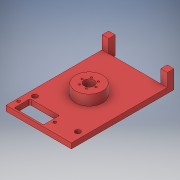
# Autodesk Inventor part: 000.801 - Опора
Saved by Autodesk Inventor 2019 (Build 230136000, 136)
## iProperties
Created: 2020-03-13
Part Number: 000.801 - Опора
Material: Пластик АБС
Document SubType Name: Modeling
Designer: Петров Иван
Density: 1.06 g/cm^3
Appearance: Гладкий — красный
Author: Петров Иван
Autodesk Inventor part; units mm, degrees
ref_plane "YZ Plane" through (0, 0, 0) normal (1, 0, 0) x (0, 1, 0)
ref_plane "XZ Plane" through (0, 0, 0) normal (0, 1, 0) x (-1, 0, 0)
ref_plane "XY Plane" through (0, 0, 0) normal (0, 0, 1) x (1, 0, 0)
sketch "Эскиз1" plane through (0, 0, 0) normal (0, 1, 0) x (-1, 0, 0)
  circle A0 centre (-2.65, -4.5899) radius 0.75
  circle A1 centre (2.65, -4.5899) radius 0.75
  circle A2 centre (5.3, 0) radius 0.75
  circle A3 centre (2.65, 4.5899) radius 0.75
  circle A4 centre (-2.65, 4.5899) radius 0.75
  circle A5 centre (-5.3, 0) radius 0.75
  circle A6 centre (0, 0) radius 3.85
  arc A7 (-3.4059, 8.2225) -> (-3.1756, 6.1003) centre (3.6513, 7.9146) ccw
  arc A8 (-3.1756, 6.1003) -> (-3.6952, 5.8003) centre (0, 0) ccw
  arc A9 (-3.6952, 5.8003) -> (-5.418, 7.0608) centre (-8.6799, 0.7952) ccw
  arc A10 (-5.418, 7.0608) -> (-6.0128, 6.5618) centre (0, 0) ccw
  arc A11 (-6.0128, 6.5618) -> (-5.0705, 4.6463) centre (0.7241, 8.6861) ccw
  arc A12 (-5.0705, 4.6463) -> (-5.4562, 4.1867) centre (0, 0) ccw
  arc A13 (-5.4562, 4.1867) -> (-7.5062, 4.782) centre (-8.4284, -2.2214) ccw
  arc A14 (-7.5062, 4.782) -> (-7.8944, 4.1096) centre (0, 0) ccw
  arc A15 (-7.8944, 4.1096) -> (-6.3539, 2.6319) centre (-2.2904, 8.4099) ccw
  arc A16 (-6.3539, 2.6319) -> (-6.5591, 2.0681) centre (0, 0) ccw
  arc A17 (-6.5591, 2.0681) -> (-8.689, 1.9263) centre (-7.1604, -4.9702) ccw
  arc A18 (-8.689, 1.9263) -> (-8.8239, 1.1617) centre (0, 0) ccw
  arc A19 (-8.8239, 1.1617) -> (-6.8708, 0.3) centre (-5.0286, 7.1194) ccw
  arc A20 (-6.8708, 0.3) -> (-6.8708, -0.3) centre (0, 0) ccw
  arc A21 (-6.8708, -0.3) -> (-8.8239, -1.1617) centre (-5.0286, -7.1194) ccw
  arc A22 (-8.8239, -1.1617) -> (-8.689, -1.9263) centre (0, 0) ccw
  arc A23 (-8.689, -1.9263) -> (-6.5591, -2.0681) centre (-7.1604, 4.9702) ccw
  arc A24 (-6.5591, -2.0681) -> (-6.3539, -2.6319) centre (0, 0) ccw
  arc A25 (-6.3539, -2.6319) -> (-7.8944, -4.1096) centre (-2.2904, -8.4099) ccw
  arc A26 (-7.8944, -4.1096) -> (-7.5062, -4.782) centre (0, 0) ccw
  arc A27 (-7.5062, -4.782) -> (-5.4562, -4.1867) centre (-8.4284, 2.2214) ccw
  arc A28 (-5.4562, -4.1867) -> (-5.0705, -4.6463) centre (0, 0) ccw
  arc A29 (-5.0705, -4.6463) -> (-6.0128, -6.5618) centre (0.7241, -8.6861) ccw
  arc A30 (-6.0128, -6.5618) -> (-5.418, -7.0608) centre (0, 0) ccw
  arc A31 (-5.418, -7.0608) -> (-3.6952, -5.8003) centre (-8.6799, -0.7952) ccw
  arc A32 (-3.6952, -5.8003) -> (-3.1756, -6.1003) centre (0, 0) ccw
  arc A33 (-3.1756, -6.1003) -> (-3.4059, -8.2225) centre (3.6513, -7.9146) ccw
  arc A34 (-3.4059, -8.2225) -> (-2.6763, -8.4881) centre (0, 0) ccw
  arc A35 (-2.6763, -8.4881) -> (-1.4885, -6.7144) centre (-7.8845, -3.716) ccw
  arc A36 (-1.4885, -6.7144) -> (-0.8977, -6.8185) centre (0, 0) ccw
  arc A37 (-0.8977, -6.8185) -> (-0.3882, -8.8915) centre (6.138, -6.1885) ccw
  arc A38 (-0.3882, -8.8915) -> (0.3882, -8.8915) centre (0, 0) ccw
  arc A39 (0.3882, -8.8915) -> (0.8977, -6.8185) centre (-6.138, -6.1885) ccw
  arc A40 (0.8977, -6.8185) -> (1.4885, -6.7144) centre (0, 0) ccw
  arc A41 (1.4885, -6.7144) -> (2.6763, -8.4881) centre (7.8845, -3.716) ccw
  arc A42 (2.6763, -8.4881) -> (3.4059, -8.2225) centre (0, 0) ccw
  arc A43 (3.4059, -8.2225) -> (3.1756, -6.1003) centre (-3.6513, -7.9146) ccw
  arc A44 (3.1756, -6.1003) -> (3.6952, -5.8003) centre (0, 0) ccw
  arc A45 (3.6952, -5.8003) -> (5.418, -7.0608) centre (8.6799, -0.7952) ccw
  arc A46 (5.418, -7.0608) -> (6.0128, -6.5618) centre (0, 0) ccw
  arc A47 (6.0128, -6.5618) -> (5.0705, -4.6463) centre (-0.7241, -8.6861) ccw
  arc A48 (5.0705, -4.6463) -> (5.4562, -4.1867) centre (0, 0) ccw
  arc A49 (5.4562, -4.1867) -> (7.5062, -4.782) centre (8.4284, 2.2214) ccw
  arc A50 (7.5062, -4.782) -> (7.8944, -4.1096) centre (0, 0) ccw
  arc A51 (7.8944, -4.1096) -> (6.3539, -2.6319) centre (2.2904, -8.4099) ccw
  arc A52 (6.3539, -2.6319) -> (6.5591, -2.0681) centre (0, 0) ccw
  arc A53 (6.5591, -2.0681) -> (8.689, -1.9263) centre (7.1604, 4.9702) ccw
  arc A54 (8.689, -1.9263) -> (8.8239, -1.1617) centre (0, 0) ccw
  arc A55 (8.8239, -1.1617) -> (6.8708, -0.3) centre (5.0286, -7.1194) ccw
  arc A56 (6.8708, -0.3) -> (6.8708, 0.3) centre (0, 0) ccw
  arc A57 (6.8708, 0.3) -> (8.8239, 1.1617) centre (5.0286, 7.1194) ccw
  arc A58 (8.8239, 1.1617) -> (8.689, 1.9263) centre (0, 0) ccw
  arc A59 (8.689, 1.9263) -> (6.5591, 2.0681) centre (7.1604, -4.9702) ccw
  arc A60 (6.5591, 2.0681) -> (6.3539, 2.6319) centre (0, 0) ccw
  arc A61 (6.3539, 2.6319) -> (7.8944, 4.1096) centre (2.2904, 8.4099) ccw
  arc A62 (7.8944, 4.1096) -> (7.5062, 4.782) centre (0, 0) ccw
  arc A63 (7.5062, 4.782) -> (5.4562, 4.1867) centre (8.4284, -2.2214) ccw
  arc A64 (5.4562, 4.1867) -> (5.0705, 4.6463) centre (0, 0) ccw
  arc A65 (5.0705, 4.6463) -> (6.0128, 6.5618) centre (-0.7241, 8.6861) ccw
  arc A66 (6.0128, 6.5618) -> (5.418, 7.0608) centre (0, 0) ccw
  arc A67 (5.418, 7.0608) -> (3.6952, 5.8003) centre (8.6799, 0.7952) ccw
  arc A68 (3.6952, 5.8003) -> (3.1756, 6.1003) centre (0, 0) ccw
  arc A69 (3.1756, 6.1003) -> (3.4059, 8.2225) centre (-3.6513, 7.9146) ccw
  arc A70 (3.4059, 8.2225) -> (2.6763, 8.4881) centre (0, 0) ccw
  arc A71 (2.6763, 8.4881) -> (1.4885, 6.7144) centre (7.8845, 3.716) ccw
  arc A72 (1.4885, 6.7144) -> (0.8977, 6.8185) centre (0, 0) ccw
  arc A73 (0.8977, 6.8185) -> (0.3882, 8.8915) centre (-6.138, 6.1885) ccw
  arc A74 (0.3882, 8.8915) -> (-0.3882, 8.8915) centre (0, 0) ccw
  arc A75 (-0.3882, 8.8915) -> (-0.8977, 6.8185) centre (6.138, 6.1885) ccw
  arc A76 (-0.8977, 6.8185) -> (-1.4885, 6.7144) centre (0, 0) ccw
  arc A77 (-1.4885, 6.7144) -> (-2.6763, 8.4881) centre (-7.8845, 3.716) ccw
  arc A78 (-2.6763, 8.4881) -> (-3.4059, 8.2225) centre (0, 0) ccw
  line L0 (-25, 25) -> (25, 25)
  line L1 (25, 25) -> (25, -25)
  line L2 (25, -25) -> (-25, -25)
  line L3 (-25, -25) -> (-25, 25)
  line L4 (-25, 25) -> (25, -25) construction
  line L5 (25, 25) -> (-25, -25) construction
  dimension "d4" = 50
  dimension "d5" = 50
  constraints: 144 point on circle, 79 centre point, 12 end point, 2 midpoint, 2 parallel, 1 horizontal, 1 perpendicular
  measures "d4" distance of L1.end L2.end
  measures "d5" distance of L0.end L1.end
extrude "Выдавливание1" add sketch "Эскиз1" along normal blind 4 contours A78 A77 A76 A75 A74 A73 A72 A71 A70 A69 A68 A67 A66 A65 A64 A63 A62 A61 A60 A59 A58 A57 A56 A55 A54 A53 A52 A51 A50 A49 A48 A47 A46 A45 A44 A43 A42 A41 A40 A39 A38 A37 A36 A35 A34 A33 A32 A31 A30 A29 A28 A27 A26 A25 A24 A23 A22 A21 A20 A19 A18 A17 A16 A15 A14 A13 A12 A11 A10 A9 A8 A7 | L0 L1 L2 L3
sketch "Эскиз2" plane through (0, 4, 0) normal (0, 1, 0) x (1, 0, 0)
  line L0 (-8.6363, -28.2584) -> (-8.5162, -28.2584)
  arc A0 (-8.5162, -34.0584) -> (-8.5162, -28.2584) centre (-8.5162, -31.1584) ccw
  line L1 (-8.5162, -34.0584) -> (-8.6363, -34.0584)
  arc A1 (-12.5542, -37.1584) -> (-8.6363, -34.0584) centre (-14.1162, -31.1584) ccw
  line L2 (-12.5542, -37.1584) -> (1.4338, -37.1584)
  arc A2 (1.4338, -37.1584) -> (2.1838, -36.4084) centre (1.4338, -36.4084) ccw
  line L3 (2.1838, -36.4084) -> (2.1838, -25.9084)
  arc A3 (2.1838, -25.9084) -> (1.4338, -25.1584) centre (1.4338, -25.9084) ccw
  line L4 (1.4338, -25.1584) -> (-12.5542, -25.1584)
  arc A4 (-8.6363, -28.2584) -> (-12.5542, -25.1584) centre (-14.1162, -31.1584) ccw
  line L5 (-4.2162, -36.2584) -> (0.7838, -36.2584)
  arc A5 (-4.7162, -35.7584) -> (-4.2162, -36.2584) centre (-4.2162, -35.7584) ccw
  line L6 (-4.7162, -26.5584) -> (-4.7162, -35.7584)
  arc A6 (-4.2162, -26.0584) -> (-4.7162, -26.5584) centre (-4.2162, -26.5584) ccw
  line L7 (0.7838, -26.0584) -> (-4.2162, -26.0584)
  arc A7 (1.2838, -26.5584) -> (0.7838, -26.0584) centre (0.7838, -26.5584) ccw
  line L8 (1.2838, -35.7584) -> (1.2838, -26.5584)
  arc A8 (0.7838, -36.2584) -> (1.2838, -35.7584) centre (0.7838, -35.7584) ccw
  arc A9 (5.8864, -30.6084) -> (5.8864, -31.7084) centre (4.9338, -31.1584) ccw
  line L9 (7.0838, -30.6084) -> (5.8864, -30.6084)
  line L10 (7.0838, -30.6084) -> (7.0838, -25.9084)
  arc A10 (7.0838, -25.9084) -> (6.2338, -25.0584) centre (6.2338, -25.9084) ccw
  line L11 (6.2338, -25.0584) -> (1.4338, -25.0584)
  arc A11 (2.2838, -25.9084) -> (1.4338, -25.0584) centre (1.4338, -25.9084) ccw
  line L12 (2.2838, -36.4084) -> (2.2838, -25.9084)
  arc A12 (1.4338, -37.2584) -> (2.2838, -36.4084) centre (1.4338, -36.4084) ccw
  line L13 (1.4338, -37.2584) -> (6.2338, -37.2584)
  arc A13 (6.2338, -37.2584) -> (7.0838, -36.4084) centre (6.2338, -36.4084) ccw
  line L14 (7.0838, -36.4084) -> (7.0838, -31.7084)
  line L15 (5.8864, -31.7084) -> (7.0838, -31.7084)
  line L16 (-25.0162, -25.9084) -> (-25.0162, -30.6084)
  line L17 (-23.8188, -30.6084) -> (-25.0162, -30.6084)
  arc A14 (-23.8188, -31.7084) -> (-23.8188, -30.6084) centre (-22.8662, -31.1584) ccw
  line L18 (-25.0162, -31.7084) -> (-23.8188, -31.7084)
  line L19 (-25.0162, -31.7084) -> (-25.0162, -36.4084)
  arc A15 (-25.0162, -36.4084) -> (-24.1662, -37.2584) centre (-24.1662, -36.4084) ccw
  line L20 (-24.1662, -37.2584) -> (-19.3662, -37.2584)
  arc A16 (-20.2162, -36.4084) -> (-19.3662, -37.2584) centre (-19.3662, -36.4084) ccw
  line L21 (-20.2162, -25.9084) -> (-20.2162, -36.4084)
  arc A17 (-19.3662, -25.0584) -> (-20.2162, -25.9084) centre (-19.3662, -25.9084) ccw
  line L22 (-19.3662, -25.0584) -> (-24.1662, -25.0584)
  arc A18 (-24.1662, -25.0584) -> (-25.0162, -25.9084) centre (-24.1662, -25.9084) ccw
  line L23 (-19.3662, -25.0584) -> (-15.6783, -25.0584)
  line L24 (-12.5542, -25.0584) -> (-14.1162, -25.0584)
  line L25 (-14.1162, -25.0584) -> (-15.6783, -25.0584)
  line L26 (-12.5542, -25.0584) -> (1.4338, -25.0584)
  line L27 (1.4338, -37.2584) -> (-12.5542, -37.2584)
  line L28 (-15.6783, -37.2584) -> (-19.3662, -37.2584)
  line L29 (-15.6783, -37.2584) -> (-14.1162, -37.2584)
  line L30 (-14.1162, -37.2584) -> (-12.5542, -37.2584)
  arc A19 (-15.6783, -25.1584) -> (-20.1162, -29.5963) centre (-14.1162, -31.1584) ccw
  line L31 (-15.6783, -25.1584) -> (-19.3662, -25.1584)
  arc A20 (-19.3662, -25.1584) -> (-20.1162, -25.9084) centre (-19.3662, -25.9084) ccw
  line L32 (-20.1162, -25.9084) -> (-20.1162, -29.5963)
  line L33 (-19.3662, -37.1584) -> (-15.6783, -37.1584)
  arc A21 (-20.1162, -32.7204) -> (-15.6783, -37.1584) centre (-14.1162, -31.1584) ccw
  line L34 (-20.1162, -32.7204) -> (-20.1162, -36.4084)
  arc A22 (-20.1162, -36.4084) -> (-19.3662, -37.1584) centre (-19.3662, -36.4084) ccw
  circle A23 centre (4.9338, -31.1584) radius 1.1
  line L35 (5.8864, -30.6084) -> (7.0838, -30.6084)
  line L36 (7.0838, -31.7084) -> (7.0838, -30.6084)
  circle A24 centre (-22.8662, -31.1584) radius 1.1
  line L37 (-25.0162, -30.6084) -> (-23.8188, -30.6084)
  line L38 (-25.0162, -31.7084) -> (-25.0162, -30.6084)
  circle A25 centre (-14.1162, -31.1584) radius 0.8
  line L39 (-25, -25) -> (-25, 25) projected
  line L40 (25, -38.5621) -> (-25, -38.5621)
  line L41 (-25, -38.5621) -> (-25, -25)
  line L42 (-25, -25) -> (25, -25)
  line L43 (25, -25) -> (25, -38.5621)
  point P0 (0, 0)
  point P1 (-8.9662, -31.1584)
  constraints: 86 end point, 46 point on circle, 25 centre point, 2 coincident, 2 parallel, 1 collinear, 1 concentric, 1 horizontal, 1 perpendicular, 1 vertical, 3 other
extrude "Выдавливание2" add sketch "Эскиз2" against normal blind 4 contours A9 L15 L14 A13 L13 A12 L12 A11 L11 A10 L10 L9 | L9 L36 L15 A23 | L10 A10 L11 L26 L24 L25 L23 L22 A18 L41 L42 L43 L40 A15 L20 L28 L29 L30 L27 L13 A13 L14 L36 | A17 L21 A16 L20 A15 L41 L18 A14 L17 A18 L22 | L17 A24 L18 L41
sketch "Эскиз3" plane through (0, 4, 0) normal (0, 1, 0) x (1, 0, 0)
  circle A0 centre (-2.65, -4.5899) radius 0.75
  circle A1 centre (2.65, -4.5899) radius 0.75
  circle A2 centre (5.3, 0) radius 0.75
  circle A3 centre (2.65, 4.5899) radius 0.75
  circle A4 centre (-2.65, 4.5899) radius 0.75
  circle A5 centre (-5.3, 0) radius 0.75
  circle A6 centre (0, 0) radius 3.85
  arc A7 (-3.4059, 8.2225) -> (-3.1756, 6.1003) centre (3.6513, 7.9146) ccw
  arc A8 (-3.1756, 6.1003) -> (-3.6952, 5.8003) centre (0, 0) ccw
  arc A9 (-3.6952, 5.8003) -> (-5.418, 7.0608) centre (-8.6799, 0.7952) ccw
  arc A10 (-5.418, 7.0608) -> (-6.0128, 6.5618) centre (0, 0) ccw
  arc A11 (-6.0128, 6.5618) -> (-5.0705, 4.6463) centre (0.7241, 8.6861) ccw
  arc A12 (-5.0705, 4.6463) -> (-5.4562, 4.1867) centre (0, 0) ccw
  arc A13 (-5.4562, 4.1867) -> (-7.5062, 4.782) centre (-8.4284, -2.2214) ccw
  arc A14 (-7.5062, 4.782) -> (-7.8944, 4.1096) centre (0, 0) ccw
  arc A15 (-7.8944, 4.1096) -> (-6.3539, 2.6319) centre (-2.2904, 8.4099) ccw
  arc A16 (-6.3539, 2.6319) -> (-6.5591, 2.0681) centre (0, 0) ccw
  arc A17 (-6.5591, 2.0681) -> (-8.689, 1.9263) centre (-7.1604, -4.9702) ccw
  arc A18 (-8.689, 1.9263) -> (-8.8239, 1.1617) centre (0, 0) ccw
  arc A19 (-8.8239, 1.1617) -> (-6.8708, 0.3) centre (-5.0286, 7.1194) ccw
  arc A20 (-6.8708, 0.3) -> (-6.8708, -0.3) centre (0, 0) ccw
  arc A21 (-6.8708, -0.3) -> (-8.8239, -1.1617) centre (-5.0286, -7.1194) ccw
  arc A22 (-8.8239, -1.1617) -> (-8.689, -1.9263) centre (0, 0) ccw
  arc A23 (-8.689, -1.9263) -> (-6.5591, -2.0681) centre (-7.1604, 4.9702) ccw
  arc A24 (-6.5591, -2.0681) -> (-6.3539, -2.6319) centre (0, 0) ccw
  arc A25 (-6.3539, -2.6319) -> (-7.8944, -4.1096) centre (-2.2904, -8.4099) ccw
  arc A26 (-7.8944, -4.1096) -> (-7.5062, -4.782) centre (0, 0) ccw
  arc A27 (-7.5062, -4.782) -> (-5.4562, -4.1867) centre (-8.4284, 2.2214) ccw
  arc A28 (-5.4562, -4.1867) -> (-5.0705, -4.6463) centre (0, 0) ccw
  arc A29 (-5.0705, -4.6463) -> (-6.0128, -6.5618) centre (0.7241, -8.6861) ccw
  arc A30 (-6.0128, -6.5618) -> (-5.418, -7.0608) centre (0, 0) ccw
  arc A31 (-5.418, -7.0608) -> (-3.6952, -5.8003) centre (-8.6799, -0.7952) ccw
  arc A32 (-3.6952, -5.8003) -> (-3.1756, -6.1003) centre (0, 0) ccw
  arc A33 (-3.1756, -6.1003) -> (-3.4059, -8.2225) centre (3.6513, -7.9146) ccw
  arc A34 (-3.4059, -8.2225) -> (-2.6763, -8.4881) centre (0, 0) ccw
  arc A35 (-2.6763, -8.4881) -> (-1.4885, -6.7144) centre (-7.8845, -3.716) ccw
  arc A36 (-1.4885, -6.7144) -> (-0.8977, -6.8185) centre (0, 0) ccw
  arc A37 (-0.8977, -6.8185) -> (-0.3882, -8.8915) centre (6.138, -6.1885) ccw
  arc A38 (-0.3882, -8.8915) -> (0.3882, -8.8915) centre (0, 0) ccw
  arc A39 (0.3882, -8.8915) -> (0.8977, -6.8185) centre (-6.138, -6.1885) ccw
  arc A40 (0.8977, -6.8185) -> (1.4885, -6.7144) centre (0, 0) ccw
  arc A41 (1.4885, -6.7144) -> (2.6763, -8.4881) centre (7.8845, -3.716) ccw
  arc A42 (2.6763, -8.4881) -> (3.4059, -8.2225) centre (0, 0) ccw
  arc A43 (3.4059, -8.2225) -> (3.1756, -6.1003) centre (-3.6513, -7.9146) ccw
  arc A44 (3.1756, -6.1003) -> (3.6952, -5.8003) centre (0, 0) ccw
  arc A45 (3.6952, -5.8003) -> (5.418, -7.0608) centre (8.6799, -0.7952) ccw
  arc A46 (5.418, -7.0608) -> (6.0128, -6.5618) centre (0, 0) ccw
  arc A47 (6.0128, -6.5618) -> (5.0705, -4.6463) centre (-0.7241, -8.6861) ccw
  arc A48 (5.0705, -4.6463) -> (5.4562, -4.1867) centre (0, 0) ccw
  arc A49 (5.4562, -4.1867) -> (7.5062, -4.782) centre (8.4284, 2.2214) ccw
  arc A50 (7.5062, -4.782) -> (7.8944, -4.1096) centre (0, 0) ccw
  arc A51 (7.8944, -4.1096) -> (6.3539, -2.6319) centre (2.2904, -8.4099) ccw
  arc A52 (6.3539, -2.6319) -> (6.5591, -2.0681) centre (0, 0) ccw
  arc A53 (6.5591, -2.0681) -> (8.689, -1.9263) centre (7.1604, 4.9702) ccw
  arc A54 (8.689, -1.9263) -> (8.8239, -1.1617) centre (0, 0) ccw
  arc A55 (8.8239, -1.1617) -> (6.8708, -0.3) centre (5.0286, -7.1194) ccw
  arc A56 (6.8708, -0.3) -> (6.8708, 0.3) centre (0, 0) ccw
  arc A57 (6.8708, 0.3) -> (8.8239, 1.1617) centre (5.0286, 7.1194) ccw
  arc A58 (8.8239, 1.1617) -> (8.689, 1.9263) centre (0, 0) ccw
  arc A59 (8.689, 1.9263) -> (6.5591, 2.0681) centre (7.1604, -4.9702) ccw
  arc A60 (6.5591, 2.0681) -> (6.3539, 2.6319) centre (0, 0) ccw
  arc A61 (6.3539, 2.6319) -> (7.8944, 4.1096) centre (2.2904, 8.4099) ccw
  arc A62 (7.8944, 4.1096) -> (7.5062, 4.782) centre (0, 0) ccw
  arc A63 (7.5062, 4.782) -> (5.4562, 4.1867) centre (8.4284, -2.2214) ccw
  arc A64 (5.4562, 4.1867) -> (5.0705, 4.6463) centre (0, 0) ccw
  arc A65 (5.0705, 4.6463) -> (6.0128, 6.5618) centre (-0.7241, 8.6861) ccw
  arc A66 (6.0128, 6.5618) -> (5.418, 7.0608) centre (0, 0) ccw
  arc A67 (5.418, 7.0608) -> (3.6952, 5.8003) centre (8.6799, 0.7952) ccw
  arc A68 (3.6952, 5.8003) -> (3.1756, 6.1003) centre (0, 0) ccw
  arc A69 (3.1756, 6.1003) -> (3.4059, 8.2225) centre (-3.6513, 7.9146) ccw
  arc A70 (3.4059, 8.2225) -> (2.6763, 8.4881) centre (0, 0) ccw
  arc A71 (2.6763, 8.4881) -> (1.4885, 6.7144) centre (7.8845, 3.716) ccw
  arc A72 (1.4885, 6.7144) -> (0.8977, 6.8185) centre (0, 0) ccw
  arc A73 (0.8977, 6.8185) -> (0.3882, 8.8915) centre (-6.138, 6.1885) ccw
  arc A74 (0.3882, 8.8915) -> (-0.3882, 8.8915) centre (0, 0) ccw
  arc A75 (-0.3882, 8.8915) -> (-0.8977, 6.8185) centre (6.138, 6.1885) ccw
  arc A76 (-0.8977, 6.8185) -> (-1.4885, 6.7144) centre (0, 0) ccw
  arc A77 (-1.4885, 6.7144) -> (-2.6763, 8.4881) centre (-7.8845, 3.716) ccw
  arc A78 (-2.6763, 8.4881) -> (-3.4059, 8.2225) centre (0, 0) ccw
  line L0 (-25, 25) -> (25, 25)
  line L1 (25, 25) -> (25, -25)
  circle A79 centre (0, 0) radius 10.4315
  dimension "d9" = 50
  constraints: 144 point on circle, 80 centre point, 4 end point, 1 coincident, 1 horizontal, 1 perpendicular
  measures "d9" distance of L0.end L1.end
extrude "Выдавливание3" add sketch "Эскиз3" along normal blind 8 contours A78 A77 A76 A75 A74 A73 A72 A71 A70 A69 A68 A67 A66 A65 A64 A63 A62 A61 A60 A59 A58 A57 A56 A55 A54 A53 A52 A51 A50 A49 A48 A47 A46 A45 A44 A43 A42 A41 A40 A39 A38 A37 A36 A35 A34 A33 A32 A31 A30 A29 A28 A27 A26 A25 A24 A23 A22 A21 A20 A19 A18 A17 A16 A15 A14 A13 A12 A11 A10 A9 A8 A7 | A79
sketch "Эскиз5" plane through (0, 0, 0) normal (0, -1, 0) x (1, 0, 0)
  circle A0 centre (20, 28.5584) radius 2 projected
  circle A1 centre (-20, 21.5621) radius 2
  line L0 (25, 38.5621) -> (-25, 38.5621) projected
  point P0 (0, 0)
  dimension "d15" = 17
  constraints: 1 centre point
  measures "d15" distance from line of L0 A1.centre
extrude "Выдавливание4" cut sketch "Эскиз5" against normal blind 12.25
move faces "Перенос1" translate (0, 0, -10) faces at (-8.3333, 1.3333, -25)
sketch "Эскиз6" plane through (0, 4, 0) normal (0, 1, 0) x (1, 0, 0)
  line L0 (25, 35) -> (-25, 35) projected
  line L1 (-25, 35) -> (-20, 35)
  line L2 (-20, 35) -> (-20, 40)
  line L3 (-20, 40) -> (-25, 40)
  line L4 (-25, 40) -> (-25, 35)
  line L5 (25, 35) -> (20, 35)
  line L6 (20, 35) -> (20, 40)
  line L7 (20, 40) -> (25, 40)
  line L8 (25, 40) -> (25, 35)
  point P0 (0, 0)
  dimension "d19" = 5
  dimension "d20" = 5
  dimension "d21" = 5
  dimension "d22" = 5
  constraints: 16 end point, 4 parallel, 2 horizontal, 2 perpendicular
  measures "d19" distance of L3.end L2.end
  measures "d20" distance of L2.end L1.end
  measures "d21" distance of L6.end L7.end
  measures "d22" distance of L5.end L6.end
extrude "Выдавливание5" add sketch "Эскиз6" along normal blind 10 and the other way blind 4
